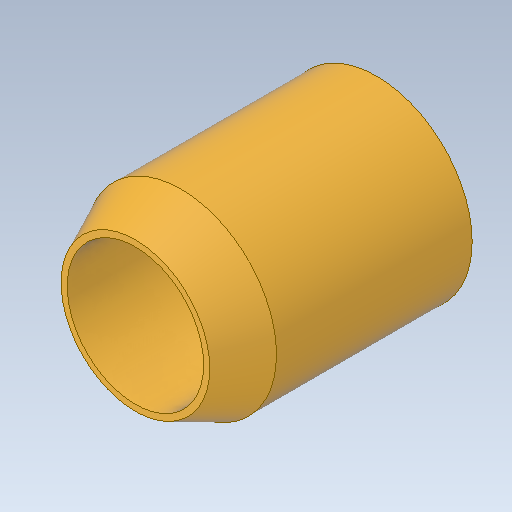
# Autodesk Inventor part: Nikon-Objective-Insulation
Saved by Autodesk Inventor 2020.5 (Build 245400000, 400)
## iProperties
Created: 2018-11-08
Part Number: Nikon-Objective-Insulation
Material: ABS Plastic
Document SubType Name: Modeling
Designer: rainer
Density: 1.06 g/cm^3
Appearance: Smooth - White
Author: rainer
Autodesk Inventor part; units mm, degrees
ref_plane "YZ Plane" through (0, 0, 0) normal (1, 0, 0) x (0, 1, 0)
ref_plane "XZ Plane" through (0, 0, 0) normal (0, 1, 0) x (-1, 0, 0)
ref_plane "XY Plane" through (0, 0, 0) normal (0, 0, 1) x (1, 0, 0)
sketch "Sketch1" plane through (0, 0, 0) normal (0, 0, 1) x (1, 0, 0)
  circle A0 centre (0, 0) radius 15
  circle A1 centre (0, 0) radius 21
  dimension "d0" = 30
  dimension "d1" = 42
  constraints: 2 centre point, 2 coincident
  measures "d0" diameter of A0
  measures "d1" diameter of A1
extrude "Extrusion1" add sketch "Sketch1" along normal blind 53
sketch "Sketch2" plane through (0, 0, 0) normal (0, 0, -1) x (-1, 0, 0)
  circle A0 centre (0, 0) radius 17.5
  circle A1 centre (0, 0) radius 21
  dimension "d4" = 35
  dimension "d5" = 42
  constraints: 2 centre point, 2 coincident
  measures "d4" diameter of A0
  measures "d5" diameter of A1
extrude "Extrusion2" add sketch "Sketch2" along normal blind 5
chamfer "Chamfer2" distance 10 angle 25 1 edges at (-21, 0, 53) measured on face at (20.9319, -1.6898, 35.3333)
thicken "Thicken1" operation add thickness 5 both sides no extend neighbours yes toward (0, 0, 1) faces at (-19.4604, -3.0712, -5)
body "Solid1"
